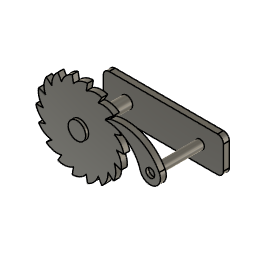
paw and ratchet v1 (Autodesk Fusion 360 design; units mm, degrees)
Autodesk Fusion 360 part; units mm, degrees
note: some values were not read from the file. Set by a fixed rule: which sketch regions a step uses.
sketch "Sketch1" plane through (0, 0, 0) normal (0, 1, 0) x (1, 0, 0) in component "ratchet"
  circle A0 centre (0, 0) radius 62.5
  circle A1 centre (0, 0) radius 10
  circle A2 centre (0, 0) radius 15
  circle A3 centre (0, 0) radius 75
  line L0 (0, 0) -> (13.0236, -73.8606)
  line L1 (0, 0) -> (75, 0) construction
  line L2 (0, 0) -> (-10.853, -61.5505)
  arc A4 (-10.853, -61.5505) -> (13.0236, -73.8606) centre (13.378, -43.8627) ccw
  dimension "d1" = 125
  dimension "d2" = 20
  dimension "d3" = 30
  dimension "d4" = 12.5
  dimension "d5" = 80
  dimension "d6" = 20
  dimension "d7" = 30
  constraint coincident A0.centre A1.centre
  constraint concentric A1 A2
  constraint horizontal L1
  constraint coincident A0 L2.end
  constraint coincident A3 L0.end
  measures "d1" diameter of A0
  measures "d2" diameter of A1
  measures "d3" diameter of A2
  measures "d5" angle of L0 L1
  measures "d6" angle of L0 L2
  measures "d7" radius of A4
extrude "Extrude1" add sketch "Sketch1" along normal mid plane 10 contours A0 A2 L0 L2 | A0 L0 A4 picked at (5.1197, -46.3065) makes body 1 in component "ratchet"
pattern_circular "C-Pattern1" count 18 over 360 about axis through (0, -5, 0) along (0, 1, 0) of bodies 1 makes body 2 at (18.6177, 5, 46.4976) makes body 3 at (33.398, -5, 37.3258) makes body 4 at (44.15, 5, 23.652) makes body 5 at (49.5769, 5, 7.1254) makes body 6 at (49.0241, 5, -10.2606) makes body 7 at (42.5583, 5, -26.409) makes body 8 at (30.9593, 5, -39.3722) makes body 9 at (15.6261, 5, -47.5864) makes body 10 at (-1.5918, 5, -50.0611) makes body 11 at (-18.6177, 5, -46.4976) makes body 12 at (-33.398, 5, -37.3258) makes body 13 at (-44.15, 5, -23.652) makes body 14 at (-49.5769, 5, -7.1254) makes body 15 at (-49.0241, 5, 10.2606) makes body 16 at (-42.5583, 5, 26.409) makes body 17 at (-30.9593, 5, 39.3722) makes body 18 at (-15.6261, 5, 47.5864) in component "ratchet"
extrude "Extrude2" add sketch "Sketch1" along normal mid plane 20 contours A1 A2 L0 L2 | A1 A2 L0 L2 bodies 1 2 3 4 5 6 7 8 9 10 11 12 13 14 15 16 17 18 in component "ratchet"
sketch "Sketch1 (2)" plane through (0, -5, 0) normal (0, -1, 0) x (1, 0, 0) in component "paw"
  line L0 (-31.25, 54.1266) -> (-37.5, 64.9519)
  arc A0 (-37.5, 64.9519) -> (-47.8778, 40.1742) centre (-17.9462, 42.2) ccw
  line L1 (-47.8778, 40.1742) -> (-57.4533, 48.2091)
  arc A1 (-57.4533, 48.2091) -> (-58.7308, 21.3763) centre (-31.2972, 33.517) ccw
  line L2 (-58.7308, 21.3763) -> (-70.4769, 25.6515)
  arc A2 (-70.4769, 25.6515) -> (-62.5, 0) centre (-40.8732, 20.7914) ccw
  line L3 (-62.5, 0) -> (-75, 0)
  arc A3 (-75, 0) -> (-58.7308, -21.3763) centre (-45.5194, 5.5581) ccw
  line L4 (-58.7308, -21.3763) -> (-70.4769, -25.6515)
  arc A4 (-70.4769, -25.6515) -> (-47.8778, -40.1742) centre (-44.6752, -10.3457) ccw
  line L5 (-47.8778, -40.1742) -> (-57.4533, -48.2091)
  arc A5 (-57.4533, -48.2091) -> (-31.25, -54.1266) centre (-38.4425, -25.0016) ccw
  line L6 (-31.25, -54.1266) -> (-37.5, -64.9519)
  arc A6 (-37.5, -64.9519) -> (-10.853, -61.5505) centre (-27.5731, -36.6419) ccw
  line L7 (-10.853, -61.5505) -> (-13.0236, -73.8606)
  arc A7 (-13.0236, -73.8606) -> (10.853, -61.5505) centre (-13.378, -43.8627) ccw
  line L8 (10.853, -61.5505) -> (13.0236, -73.8606)
  arc A8 (13.0236, -73.8606) -> (31.25, -54.1266) centre (2.4307, -45.793) ccw
  line L9 (31.25, -54.1266) -> (37.5, -64.9519)
  arc A9 (37.5, -64.9519) -> (47.8778, -40.1742) centre (17.9462, -42.2) ccw
  line L10 (47.8778, -40.1742) -> (57.4533, -48.2091)
  arc A10 (57.4533, -48.2091) -> (58.7308, -21.3763) centre (31.2972, -33.517) ccw
  line L11 (58.7308, -21.3763) -> (70.4769, -25.6515)
  arc A11 (70.4769, -25.6515) -> (62.5, 0) centre (40.8732, -20.7914) ccw
  line L12 (62.5, 0) -> (75, 0)
  arc A12 (75, 0) -> (58.7308, 21.3763) centre (45.5194, -5.5581) ccw
  line L13 (58.7308, 21.3763) -> (70.4769, 25.6515)
  arc A13 (70.4769, 25.6515) -> (47.8778, 40.1742) centre (44.6752, 10.3457) ccw
  line L14 (47.8778, 40.1742) -> (57.4533, 48.2091)
  arc A14 (57.4533, 48.2091) -> (31.25, 54.1266) centre (38.4425, 25.0016) ccw
  line L15 (31.25, 54.1266) -> (37.5, 64.9519)
  arc A15 (37.5, 64.9519) -> (10.853, 61.5505) centre (27.5731, 36.6419) ccw
  line L16 (10.853, 61.5505) -> (13.0236, 73.8606)
  arc A16 (13.0236, 73.8606) -> (-10.853, 61.5505) centre (13.378, 43.8627) ccw
  line L17 (-10.853, 61.5505) -> (-13.0236, 73.8606)
  arc A17 (-13.0236, 73.8606) -> (-31.25, 54.1266) centre (-2.4307, 45.793) ccw
  circle A18 centre (0, 0) radius 15
  circle A19 centre (0, 0) radius 10
  line L18 (-13.0236, 73.8606) -> (-10.853, 61.5505)
  arc A20 (-13.0236, 73.8606) -> (-31.25, 54.1266) centre (-2.4307, 45.793) ccw
  line L19 (-37.5, 64.9519) -> (-31.25, 54.1266)
  arc A21 (-37.5, 64.9519) -> (-47.8778, 40.1742) centre (-17.9462, 42.2) ccw
  line L20 (-57.4533, 48.2091) -> (-47.8778, 40.1742)
  arc A22 (-57.4533, 48.2091) -> (-58.7308, 21.3763) centre (-31.2972, 33.517) ccw
  line L21 (-70.4769, 25.6515) -> (-58.7308, 21.3763)
  arc A23 (-70.4769, 25.6515) -> (-62.5, 0) centre (-40.8732, 20.7914) ccw
  line L22 (-75, 0) -> (-62.5, 0)
  arc A24 (-75, 0) -> (-58.7308, -21.3763) centre (-45.5194, 5.5581) ccw
  line L23 (-70.4769, -25.6515) -> (-58.7308, -21.3763)
  arc A25 (-70.4769, -25.6515) -> (-47.8778, -40.1742) centre (-44.6752, -10.3457) ccw
  line L24 (-57.4533, -48.2091) -> (-47.8778, -40.1742)
  arc A26 (-57.4533, -48.2091) -> (-31.25, -54.1266) centre (-38.4425, -25.0016) ccw
  line L25 (-37.5, -64.9519) -> (-31.25, -54.1266)
  arc A27 (-37.5, -64.9519) -> (-10.853, -61.5505) centre (-27.5731, -36.6419) ccw
  line L26 (-13.0236, -73.8606) -> (-10.853, -61.5505)
  arc A28 (-13.0236, -73.8606) -> (10.853, -61.5505) centre (-13.378, -43.8627) ccw
  line L27 (13.0236, -73.8606) -> (10.853, -61.5505)
  arc A29 (13.0236, -73.8606) -> (31.25, -54.1266) centre (2.4307, -45.793) ccw
  line L28 (37.5, -64.9519) -> (31.25, -54.1266)
  arc A30 (37.5, -64.9519) -> (47.8778, -40.1742) centre (17.9462, -42.2) ccw
  line L29 (57.4533, -48.2091) -> (47.8778, -40.1742)
  arc A31 (57.4533, -48.2091) -> (58.7308, -21.3763) centre (31.2972, -33.517) ccw
  line L30 (70.4769, -25.6515) -> (58.7308, -21.3763)
  arc A32 (70.4769, -25.6515) -> (62.5, 0) centre (40.8732, -20.7914) ccw
  line L31 (75, 0) -> (62.5, 0)
  arc A33 (75, 0) -> (58.7308, 21.3763) centre (45.5194, -5.5581) ccw
  line L32 (70.4769, 25.6515) -> (58.7308, 21.3763)
  arc A34 (70.4769, 25.6515) -> (47.8778, 40.1742) centre (44.6752, 10.3457) ccw
  line L33 (57.4533, 48.2091) -> (47.8778, 40.1742)
  arc A35 (57.4533, 48.2091) -> (31.25, 54.1266) centre (38.4425, 25.0016) ccw
  line L34 (37.5, 64.9519) -> (31.25, 54.1266)
  arc A36 (37.5, 64.9519) -> (10.853, 61.5505) centre (27.5731, 36.6419) ccw
  line L35 (13.0236, 73.8606) -> (10.853, 61.5505)
  arc A37 (13.0236, 73.8606) -> (-10.853, 61.5505) centre (13.378, 43.8627) ccw
  circle A38 centre (125, 0) radius 7.5
  circle A39 centre (125, 0) radius 17.5
  line L36 (47.8778, 40.1742) -> (149.9857, 40.1742) construction
  line L37 (47.8778, 40.1742) -> (56.538, 45.1742)
  arc A40 (108.2137, -4.9467) -> (47.8778, 40.1742) centre (47.8778, -22.727) ccw
  arc A41 (140.3479, 8.4078) -> (56.538, 45.1742) centre (74.5711, -27.6256) ccw
  dimension "d14" = 15
  dimension "d15" = 35
  dimension "d16" = 10
  dimension "d17" = 125
  dimension "d18" = 75
  dimension "d19" = 30
  constraint concentric A38 A39
  constraint horizontal L36
  constraint coincident A13.end L14.start
  constraint tangent L36 A40
  constraint coincident A39 A40.start
  constraint coincident A39 A41.start
  constraint horizontal A18.centre A38.centre
  constraint tangent A39 A40
  constraint tangent A39 A41
  measures "d14" diameter of A38
  measures "d15" diameter of A39
  measures "d16" distance of A13.end L37.end
  measures "d17" distance of A18.centre A38.centre
  measures "d18" radius of A41
  measures "d19" angle of L36 L37
extrude "Extrude1'" add sketch "Sketch1 (2)" along normal mid plane 10 separate body contours A39 L37 A40 A41 | A39 makes body 19 in component "paw"
sketch "Sketch1 (3)" plane through (0, -5, 0) normal (0, -1, 0) x (1, 0, 0) in component "base"
  line L0 (-31.25, 54.1266) -> (-37.5, 64.9519)
  arc A0 (-37.5, 64.9519) -> (-47.8778, 40.1742) centre (-17.9462, 42.2) ccw
  line L1 (-47.8778, 40.1742) -> (-57.4533, 48.2091)
  arc A1 (-57.4533, 48.2091) -> (-58.7308, 21.3763) centre (-31.2972, 33.517) ccw
  line L2 (-58.7308, 21.3763) -> (-70.4769, 25.6515)
  arc A2 (-70.4769, 25.6515) -> (-62.5, 0) centre (-40.8732, 20.7914) ccw
  line L3 (-62.5, 0) -> (-75, 0)
  arc A3 (-75, 0) -> (-58.7308, -21.3763) centre (-45.5194, 5.5581) ccw
  line L4 (-58.7308, -21.3763) -> (-70.4769, -25.6515)
  arc A4 (-70.4769, -25.6515) -> (-47.8778, -40.1742) centre (-44.6752, -10.3457) ccw
  line L5 (-47.8778, -40.1742) -> (-57.4533, -48.2091)
  arc A5 (-57.4533, -48.2091) -> (-31.25, -54.1266) centre (-38.4425, -25.0016) ccw
  line L6 (-31.25, -54.1266) -> (-37.5, -64.9519)
  arc A6 (-37.5, -64.9519) -> (-10.853, -61.5505) centre (-27.5731, -36.6419) ccw
  line L7 (-10.853, -61.5505) -> (-13.0236, -73.8606)
  arc A7 (-13.0236, -73.8606) -> (10.853, -61.5505) centre (-13.378, -43.8627) ccw
  line L8 (10.853, -61.5505) -> (13.0236, -73.8606)
  arc A8 (13.0236, -73.8606) -> (31.25, -54.1266) centre (2.4307, -45.793) ccw
  line L9 (31.25, -54.1266) -> (37.5, -64.9519)
  arc A9 (37.5, -64.9519) -> (47.8778, -40.1742) centre (17.9462, -42.2) ccw
  line L10 (47.8778, -40.1742) -> (57.4533, -48.2091)
  arc A10 (57.4533, -48.2091) -> (58.7308, -21.3763) centre (31.2972, -33.517) ccw
  line L11 (58.7308, -21.3763) -> (70.4769, -25.6515)
  arc A11 (70.4769, -25.6515) -> (62.5, 0) centre (40.8732, -20.7914) ccw
  line L12 (62.5, 0) -> (75, 0)
  arc A12 (75, 0) -> (58.7308, 21.3763) centre (45.5194, -5.5581) ccw
  line L13 (58.7308, 21.3763) -> (70.4769, 25.6515)
  arc A13 (70.4769, 25.6515) -> (47.8778, 40.1742) centre (44.6752, 10.3457) ccw
  line L14 (47.8778, 40.1742) -> (57.4533, 48.2091)
  arc A14 (57.4533, 48.2091) -> (31.25, 54.1266) centre (38.4425, 25.0016) ccw
  line L15 (31.25, 54.1266) -> (37.5, 64.9519)
  arc A15 (37.5, 64.9519) -> (10.853, 61.5505) centre (27.5731, 36.6419) ccw
  line L16 (10.853, 61.5505) -> (13.0236, 73.8606)
  arc A16 (13.0236, 73.8606) -> (-10.853, 61.5505) centre (13.378, 43.8627) ccw
  line L17 (-10.853, 61.5505) -> (-13.0236, 73.8606)
  arc A17 (-13.0236, 73.8606) -> (-31.25, 54.1266) centre (-2.4307, 45.793) ccw
  circle A18 centre (0, 0) radius 15
  line L18 (-30, 30) -> (155, 30)
  line L19 (165, 20) -> (165, -20)
  line L20 (155, -30) -> (-30, -30)
  line L21 (-40, -20) -> (-40, 20)
  circle A19 centre (125, 0) radius 7.5
  arc A20 (-30, 30) -> (-40, 20) centre (-30, 20) ccw
  arc A21 (-40, -20) -> (-30, -30) centre (-30, -20) ccw
  arc A22 (165, 20) -> (155, 30) centre (155, 20) ccw
  arc A23 (155, -30) -> (165, -20) centre (155, -20) ccw
  circle A24 centre (0, 0) radius 10
  dimension "d22" = 40
  dimension "d23" = 30
  dimension "d24" = 30
  dimension "d25" = 40
  dimension "d26" = 10
  constraint horizontal L18
  constraint vertical L19
  constraint horizontal L20
  constraint vertical L21
  constraint tangent L18 A20
  constraint tangent L21 A20
  constraint tangent L20 A21
  constraint tangent L21 A21
  constraint equal A20 A21
  constraint tangent L18 A22
  constraint tangent L19 A22
  constraint equal A20 A22
  constraint tangent L19 A23
  constraint tangent L20 A23
  constraint equal A20 A23
  measures "d22" distance of A18.centre L21
  measures "d23" distance of A18.centre L18
  measures "d24" distance of A18.centre L20
  measures "d25" distance of L19 A19.centre
  measures "d26" radius of A20
extrude "Extrude1''" add sketch "Sketch1 (3)" against normal blind 10 from surface at -80 separate body contours A10 L11 A11 L12 A12 L13 A13 L18 L19 L20 A22 A23 | A10 L11 A11 L12 A12 L13 A13 L18 L20 L21 A20 A21 | A18 makes body 20 in component "base"
extrude "Extrude2'" add sketch "Sketch1 (3)" against normal blind 90 separate body contours A19 | A24 makes body 21 at (9.9876, 55, -0.4985) makes body 22 at (132.4907, 55, -0.3738) in component "base"
extrude "Extrude3" add sketch "Sketch1 (3)" along normal blind 5 contours A24 bodies 1 in component "ratchet"
component "paw" placed x (1, 0, 0) y (0, 1, 0) z (0, 0, 1) at (0, 0, 0)
component "base" placed x (1, 0, 0) y (0, 1, 0) z (0, 0, 1) at (0, 0, 0)
component "ratchet" placed x (1, 0, 0) y (0, 1, 0) z (0, 0, 1) at (0, 0, 0)
